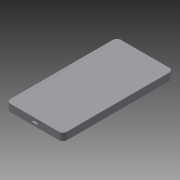
# Autodesk Inventor part: Nexus4
Saved by Autodesk Inventor 2015 (Build 190159000, 159)
## iProperties
Created: 2015-11-10
Part Number: Nexus4
Material: Generic
Document SubType Name: Modeling
Designer: Lauszus
Density: 1 g/cm^3
Appearance: Default
Author: Lauszus
Autodesk Inventor part; units mm, degrees
ref_plane "YZ Plane" through (0, 0, 0) normal (1, 0, 0) x (0, 1, 0)
ref_plane "XZ Plane" through (0, 0, 0) normal (0, 1, 0) x (-1, 0, 0)
ref_plane "XY Plane" through (0, 0, 0) normal (0, 0, 1) x (1, 0, 0)
sketch "Sketch1" plane through (0, 0, 0) normal (0, 0, 1) x (1, 0, 0)
  line L0 (-36.9502, 25.0692) -> (31.8498, 25.0692)
  line L1 (31.8498, 25.0692) -> (31.8498, -108.9308)
  line L2 (31.8498, -108.9308) -> (-36.9502, -108.9308)
  line L3 (-36.9502, -108.9308) -> (-36.9502, 25.0692)
  point P0 (0, 0)
  dimension "d0" = 68.8
  dimension "d1" = 134
  constraints: 8 end point, 2 parallel, 1 horizontal, 1 perpendicular
  measures "d0" distance of L0.start L0.end
  measures "d1" distance of L0.end L1.end
extrude "Extrusion1" add sketch "Sketch1" along normal blind 9.3
sketch "Sketch2" plane through (0, 0, 9.3) normal (0, 0, 1) x (1, 0, 0)
  line L0 (-33.5502, 9.0692) -> (28.4498, 9.0692)
  line L1 (28.4498, 9.0692) -> (28.4498, -92.4308)
  line L2 (28.4498, -92.4308) -> (-33.5502, -92.4308)
  line L3 (-33.5502, -92.4308) -> (-33.5502, 9.0692)
  line L4 (-36.9502, 25.0692) -> (-36.9502, -108.9308) projected
  line L5 (31.8498, 25.0692) -> (-36.9502, 25.0692) projected
  line L6 (-36.9502, -108.9308) -> (31.8498, -108.9308) projected
  point P0 (0, 0)
  dimension "d4" = 62
  dimension "d5" = 3.4
  dimension "d6" = 16
  dimension "d7" = 16.5
  constraints: 8 end point, 2 parallel, 1 horizontal, 1 perpendicular
  measures "d4" distance of L0.start L0.end
  measures "d5" distance between parallel lines of L4 L3
  measures "d6" distance between parallel lines of L5 L0
  measures "d7" distance between parallel lines of L6 L2
extrude "Extrusion2" cut sketch "Sketch2" against normal blind 0.1
sketch "Sketch3" plane through (-36.9502, -108.9308, 0) normal (0, -1, 0) x (1, 0, 0)
  line L0 (30.8, 5.2565) -> (38, 5.2565)
  line L1 (38, 5.2565) -> (38, 3.1565)
  line L2 (38, 3.1565) -> (30.8, 3.1565)
  line L3 (30.8, 3.1565) -> (30.8, 5.2565)
  line L4 (0, 0) -> (0, 9.3) projected
  point P0 (36.9502, 0)
  dimension "d10" = 7.2
  dimension "d11" = 2.1
  dimension "d12" = 30.8
  constraints: 8 end point, 2 parallel, 1 horizontal, 1 perpendicular
  measures "d10" distance of L1.end L2.end
  measures "d11" distance of L0.end L1.end
  measures "d12" distance between parallel lines of L4 L3
extrude "Extrusion3" cut sketch "Sketch3" against normal blind 5
fillet "Fillet1" radius 5 4 edges at (31.8498, -108.9308, 4.65) (-36.9502, -108.9308, 4.65) (31.8498, 25.0692, 4.65) (-36.9502, 25.0692, 4.65)
fillet "Fillet2" radius 0.5 16 edges at (30.3853, -107.4663, 9.3) (31.8498, -41.9308, 9.3) (30.3853, 23.6048, 9.3) (-2.5502, 25.0692, 9.3) (-35.4858, 23.6048, 9.3) (-36.9502, -41.9308, 9.3) (-35.4858, -107.4663, 9.3) (-2.5502, -108.9308, 9.3) (30.3853, -107.4663, 0) (-2.5502, -108.9308, 0) (-35.4858, -107.4663, 0) (-36.9502, -41.9308, 0) (-35.4858, 23.6048, 0) (-2.5502, 25.0692, 0) (30.3853, 23.6048, 0) (31.8498, -41.9308, 0)
body "Solid1"
